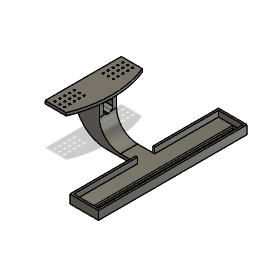
QTR-8A mount (Autodesk Fusion 360 design; units mm, degrees)
Autodesk Fusion 360 part; units mm, degrees
sketch "Sketch1" plane through (0, 0, 0) normal (0, 1, 0) x (1, 0, 0)
  circle A0 centre (0, 0) radius 52.5
  line L0 (52.5, 0) -> (37.5, 0)
  line L1 (37.5, 0) -> (48.5412, 0)
  line L2 (48.5412, 0) -> (48.5412, 20)
  line L3 (48.5412, 20) -> (37.5, 20)
  line L4 (37.5, 20) -> (37.5, 0)
  line L5 (37.5, 0) -> (48.5412, 0)
  line L6 (48.5412, 0) -> (48.5412, -20)
  line L7 (48.5412, -20) -> (37.5, -20)
  line L8 (37.5, -20) -> (37.5, 0)
  dimension "d1" = 105
  dimension "d2" = 15
  dimension "d3" = 20
  constraint coincident A0.centre origin
  constraint coincident A0 L0.start
  constraint horizontal L0
  constraint horizontal L1
  constraint vertical L2
  constraint horizontal L3
  constraint vertical L4
  constraint coincident A0 L2.end
  constraint horizontal L5
  constraint vertical L6
  constraint horizontal L7
  constraint vertical L8
  constraint coincident A0 L6.end
  measures "d1" diameter of A0
  measures "d2" distance of L0.start L0.end
  measures "d3" distance of L0.end L3.end
extrude "Extrude1" add sketch "Sketch1" along normal blind 1.5 contours A0 L0 L2 | A0 L0 L6 | L0 L1 L2 L3 L4 L5 | L0 L1 L5 L6 L7 L8 makes body 1
sketch "Sketch2" plane through (0, 1.5, 0) normal (0, 1, 0) x (-1, 0, 0)
  arc A0 (-48.5412, 20) -> (-48.5412, -20) centre (0, 0) ccw
  line L0 (-48.5412, -20) -> (-37.5, -20)
  line L1 (-37.5, -20) -> (-37.5, 20)
  line L2 (-37.5, 20) -> (-48.5412, 20)
  point P0 (-45.58, 17.78)
  point P1 (-43.04, 17.78)
  point P2 (-40.5, 17.78)
  point P3 (-45.58, 15.24)
  point P4 (-43.04, 15.24)
  point P5 (-40.5, 15.24)
  point P6 (-45.58, 12.7)
  point P7 (-43.04, 12.7)
  point P8 (-40.5, 12.7)
  point P9 (-45.58, 10.16)
  point P10 (-43.04, 10.16)
  point P11 (-40.5, 10.16)
  point P12 (-45.58, 7.62)
  point P13 (-43.04, 7.62)
  point P14 (-40.5, 7.62)
  point P15 (-45.58, -7.62)
  point P16 (-43.04, -7.62)
  point P17 (-40.5, -7.62)
  point P18 (-45.58, -10.16)
  point P19 (-43.04, -10.16)
  point P20 (-40.5, -10.16)
  point P21 (-45.58, -12.7)
  point P22 (-43.04, -12.7)
  point P23 (-40.5, -12.7)
  point P24 (-45.58, -15.24)
  point P25 (-43.04, -15.24)
  point P26 (-40.5, -15.24)
  point P27 (-45.58, -17.78)
  point P28 (-43.04, -17.78)
  point P29 (-40.5, -17.78)
  dimension "d6" = 2.54
  dimension "d7" = 2.54
  dimension "d8" = 3
  dimension "d11" = 0
  dimension "d12" = -35.56
  dimension "d13" = 2.22
  measures "d6" distance of P0 P1
  measures "d7" distance of P1 P2
  measures "d8" distance of L1 P2
  measures "d13" distance of L2 P0
hole "Hole1" at (45.58, 1.5, 17.78) at (43.04, 1.5, 17.78) at (45.58, 1.5, 15.24) at (45.58, 1.5, 12.7) at (45.58, 1.5, 10.16) at (45.58, 1.5, 7.62) at (40.5, 1.5, 7.62) at (40.5, 1.5, 10.16) at (40.5, 1.5, 17.78) at (40.5, 1.5, 15.24) at (40.5, 1.5, 12.7) at (43.04, 1.5, 10.16) at (43.04, 1.5, 15.24) at (43.04, 1.5, 7.62) at (43.04, 1.5, 12.7) at (45.58, 1.5, -10.16) at (43.04, 1.5, -10.16) at (40.5, 1.5, -10.16) at (40.5, 1.5, -17.78) at (45.58, 1.5, -7.62) at (43.04, 1.5, -15.24) at (40.5, 1.5, -7.62) at (45.58, 1.5, -12.7) at (40.5, 1.5, -15.24) at (43.04, 1.5, -12.7) at (45.58, 1.5, -17.78) at (43.04, 1.5, -7.62) at (45.58, 1.5, -15.24) at (43.04, 1.5, -17.78) at (40.5, 1.5, -12.7) direction (0, -1, 0) diameter 1 depth 9 tip angle 118 bodies 1
sketch "Sketch3" plane through (0, 0, 0) normal (0, -1, 0) x (1, 0, 0)
  circle A0 centre (43.04, -17.78) radius 0.5
  circle A1 centre (43.04, -7.62) radius 0.5
  circle A2 centre (43.04, -12.7) radius 0.5
  circle A3 centre (45.58, -12.7) radius 0.5
  circle A4 centre (43.04, -15.24) radius 0.5
  circle A5 centre (40.5, -17.78) radius 0.5
  circle A6 centre (43.04, -10.16) radius 0.5
  circle A7 centre (43.04, 12.7) radius 0.5
  circle A8 centre (43.04, 15.24) radius 0.5
  circle A9 centre (40.5, 12.7) radius 0.5
  circle A10 centre (40.5, 17.78) radius 0.5
  circle A11 centre (40.5, 7.62) radius 0.5
  circle A12 centre (45.58, 10.16) radius 0.5
  circle A13 centre (45.58, 15.24) radius 0.5
  circle A14 centre (45.58, 17.78) radius 0.5
  circle A15 centre (43.04, 17.78) radius 0.5
  circle A16 centre (45.58, 12.7) radius 0.5
  circle A17 centre (45.58, 7.62) radius 0.5
  circle A18 centre (40.5, 10.16) radius 0.5
  circle A19 centre (40.5, 15.24) radius 0.5
  circle A20 centre (43.04, 10.16) radius 0.5
  circle A21 centre (43.04, 7.62) radius 0.5
  circle A22 centre (45.58, -10.16) radius 0.5
  circle A23 centre (40.5, -10.16) radius 0.5
  circle A24 centre (45.58, -7.62) radius 0.5
  circle A25 centre (40.5, -7.62) radius 0.5
  circle A26 centre (40.5, -15.24) radius 0.5
  circle A27 centre (45.58, -17.78) radius 0.5
  circle A28 centre (45.58, -15.24) radius 0.5
  circle A29 centre (40.5, -12.7) radius 0.5
  arc A30 (48.5412, -20) -> (48.5412, 20) centre (0, 0) ccw
  line L0 (48.5412, 20) -> (37.5, 20)
  line L1 (37.5, 20) -> (37.5, -20)
  line L2 (37.5, -20) -> (48.5412, -20)
  line L3 (37.5, 0) -> (50.5, 0)
  line L4 (50.5, 0) -> (50.5, -4.5)
  line L5 (50.5, -4.5) -> (37.5, -4.5)
  line L6 (37.5, -4.5) -> (37.5, 0)
  line L7 (50.5, 0) -> (37.5, 0)
  line L8 (37.5, 0) -> (37.5, 4.5)
  line L9 (37.5, 4.5) -> (50.5, 4.5)
  line L10 (50.5, 4.5) -> (50.5, 0)
  constraint horizontal L3
  constraint vertical L4
  constraint horizontal L5
  constraint vertical L6
  constraint midpoint L1 L3.start
  constraint horizontal L7
  constraint vertical L8
  constraint horizontal L9
  constraint vertical L10
  constraint coincident L1 L8.end
extrude "Extrude2" add sketch "Sketch3" along normal blind 20 contours L1 L3 L4 L5 L6 L7 | L1 L3 L7 L8 L9 L10 bodies 1
sketch "Sketch4" plane through (50.5, 0, 0) normal (1, 0, 0) x (0, 0, -1)
  line L0 (4.5, 0) -> (-4.5, 0)
  line L1 (-4.5, 0) -> (-4.5, -20)
  line L2 (-4.5, -20) -> (4.5, -20)
  line L3 (4.5, -20) -> (4.5, 0)
  line L4 (-4.5, -20) -> (4.5, -20)
  line L5 (4.5, -20) -> (4.5, -18.5)
  line L6 (4.5, -18.5) -> (-4.5, -18.5)
  line L7 (-4.5, -18.5) -> (-4.5, -20)
  dimension "d19" = 1.5
  constraint horizontal L4
  constraint vertical L5
  constraint horizontal L6
  constraint vertical L7
  constraint coincident L1.end L2.start
  measures "d19" distance of L1.end L6.end
extrude "Extrude3" add sketch "Sketch4" along normal blind 20 contours L1 L2 L3 L4 L5 L6 L7 bodies 1
fillet "Fillet1" radius 16.5 1 edges at (37.5, -20, 0) on bodies 1
fillet "Fillet2" radius 11 1 edges at (50.5, -18.5, 0) on bodies 1
sketch "Sketch5" plane through (0, -18.5, 0) normal (0, 1, 0) x (-1, 0, 0)
  line L0 (-61.5, -4.5) -> (-61.5, 4.5)
  line L1 (-61.5, 4.5) -> (-70.5, 4.5)
  line L2 (-70.5, 4.5) -> (-70.5, -4.5)
  line L3 (-70.5, -4.5) -> (-61.5, -4.5)
  line L4 (-83.5, -38) -> (-57.5, -38)
  line L5 (-57.5, -38) -> (-57.5, 38)
  line L6 (-57.5, 38) -> (-83.5, 38)
  line L7 (-83.5, 38) -> (-83.5, -38)
  line L8 (-83.5, -38) -> (-57.5, 38) construction
  line L9 (-57.5, -38) -> (-83.5, 38) construction
  line L10 (-70.5, 0) -> (-70.5, 38)
  line L11 (-70.5, 0) -> (-70.5, -38)
  point P0 (-70.5, 0)
  dimension "d26" = 26
  dimension "d27" = 76
  constraint horizontal L4
  constraint perpendicular L4 L5
  constraint parallel L4 L6
  constraint parallel L5 L7
  constraint coincident L8 P0
  constraint coincident L9 P0
  constraint midpoint L2 P0
  constraint coincident P0 L10.start
  constraint midpoint L6 L10.end
  constraint midpoint L4 L11.end
  measures "d26" distance of L5.end L6.end
  measures "d27" distance of L4.end L5.end
extrude "Extrude4" add sketch "Sketch5" against normal blind 1.5 contours L2 L4 L6 L7 L10 L11 bodies 1
sketch "Sketch6" plane through (0, -18.5, 0) normal (0, 1, 0) x (-1, 0, 0)
  line L0 (-61.5, -4.5) -> (-61.5, 4.5)
  line L1 (-61.5, 4.5) -> (-70.5, 4.5)
  line L2 (-70.5, 4.5) -> (-70.5, 38)
  line L3 (-70.5, 38) -> (-83.5, 38)
  line L4 (-83.5, 38) -> (-83.5, -38)
  line L5 (-83.5, -38) -> (-70.5, -38)
  line L6 (-70.5, -38) -> (-70.5, -4.5)
  line L7 (-70.5, -4.5) -> (-61.5, -4.5)
  line L8 (-83.5, -38) -> (-70.5, -38)
  line L9 (-70.5, -38) -> (-70.5, 38)
  line L10 (-70.5, 38) -> (-83.5, 38)
  line L11 (-83.5, 38) -> (-83.5, -38)
  line L12 (-84.5, -39) -> (-69.5, -39)
  line L13 (-69.5, -39) -> (-69.5, 39)
  line L14 (-69.5, 39) -> (-84.5, 39)
  line L15 (-84.5, 39) -> (-84.5, -39)
  dimension "d30" = 1
  constraint horizontal L8
  constraint vertical L9
  constraint horizontal L10
  constraint vertical L11
  constraint coincident L2.end L3.start
  constraint coincident L4.end L5.start
extrude "Extrude5" add sketch "Sketch6" along normal blind 3 separate body contours L1 L2 L3 L4 L5 L6 L7 L8 L9 L10 L11 L12 L13 L14 L15 makes body 2
extrude "Extrude6" add 1 faces at (84.1667, -18.5, -12.6667) along direction (0, -1, 0) up to surface (1.5 mm away) on bodies 2 bodies 2 1
sketch "Sketch7" plane through (0, -18.5, 0) normal (0, 1, 0) x (-1, 0, 0)
  line L0 (-61.5, -4.5) -> (-61.5, 4.5)
  line L1 (-61.5, 4.5) -> (-69.5, 4.5)
  line L2 (-69.5, 4.5) -> (-70.5, 4.5)
  line L3 (-70.5, 4.5) -> (-70.5, 38)
  line L4 (-70.5, 38) -> (-83.5, 38)
  line L5 (-83.5, 38) -> (-83.5, -38)
  line L6 (-83.5, -38) -> (-70.5, -38)
  line L7 (-70.5, -38) -> (-70.5, -4.5)
  line L8 (-70.5, -4.5) -> (-69.5, -4.5)
  line L9 (-69.5, -4.5) -> (-61.5, -4.5)
  line L10 (-83.5, 38) -> (-82.6, 38)
  line L11 (-82.6, 38) -> (-82.6, 37.1)
  line L12 (-82.6, 37.1) -> (-78.6, 37.1)
  line L13 (-78.6, 37.1) -> (-78.6, -37.1)
  line L14 (-78.6, -37.1) -> (-82.6, -37.1)
  line L15 (-82.6, -37.1) -> (-82.6, 37.1)
  dimension "d35" = 0.9
  dimension "d36" = 0.9
  dimension "d37" = 4
  dimension "d38" = 0.9
  constraint coincident L4.end L5.start
  constraint perpendicular L5 L10
  constraint perpendicular L4 L11
  constraint horizontal L12
  constraint vertical L13
  constraint horizontal L14
  constraint vertical L15
  measures "d35" distance of L4.end L10.end
  measures "d36" distance of L10.end L11.end
  measures "d37" distance of L11.end L12.end
  measures "d38" distance of L6 L14
extrude "Extrude7" cut sketch "Sketch7" against normal blind 5 contours L12 L13 L14 L15 bodies 2
fillet "Fillet3" radius 0.5 4 edges at (82.6, -18.5, 0) (80.6, -18.5, 37.1) (78.6, -18.5, 0) (80.6, -18.5, -37.1) on bodies 2
sketch "Sketch8" plane through (50.5, 0, 0) normal (1, 0, 0) x (0, 0, -1)
  line L0 (-4.5, -7.5) -> (4.5, -7.5)
  line L1 (4.5, -7.5) -> (4.5, 0)
  line L2 (4.5, 0) -> (-4.5, 0)
  line L3 (-4.5, 0) -> (-4.5, -7.5)
  line L4 (2.5, -1) -> (-2.5, -1)
  line L5 (-2.5, -1) -> (-2.5, -8)
  line L6 (-2.5, -8) -> (2.5, -8)
  line L7 (2.5, -8) -> (2.5, -1)
  line L8 (2.5, -1) -> (-2.5, -8) construction
  line L9 (-2.5, -1) -> (2.5, -8) construction
  point P0 (0, -4.5)
  constraint horizontal L4
  constraint perpendicular L4 L5
  constraint parallel L4 L6
  constraint parallel L5 L7
  constraint coincident L8 P0
  constraint coincident L9 P0
extrude "Extrude8" cut sketch "Sketch8" along normal blind 1 and the other way blind 21 contours L0 L4 L5 L7 | L0 L5 L6 L7 bodies 2
fillet "Fillet4" radius 2.25 4 edges at (44, -1, -2.5) (44, -1, 2.5) (44.3184, -8, -2.5) (44.3184, -8, 2.5) on bodies 2
